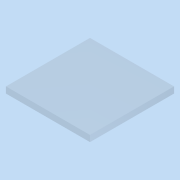
# Autodesk Inventor part: camera_hole_filter
Saved by Autodesk Inventor 2014 SP1 (Build 180222100, 222)
## iProperties
Created: 2013-03-31
Material: Glass
Document SubType Name: Modeling
Designer: Robert Davis
Mass: 1.35891 g
Surface Area: 13.4657 cm^2
Volume: 0.623352 cm^3
Density: 2.18 g/cm^3
Description: IR FILTER
Appearance: Clear - Light
Author: Robert Davis
Autodesk Inventor part; units mm, degrees
ref_plane "YZ Plane" through (0, 0, 0) normal (1, 0, 0) x (0, 1, 0)
sketch "Sketch1" plane through (0, 0, 0) normal (0, 0, 1) x (1, 0, 0)
  line L0 (0, 8.1841) -> (0, 0)
  line L1 (0, 0) -> (9.8567, 0)
  line L2 (-7.5, 7.5) -> (7.5, 7.5)
  line L3 (7.5, 7.5) -> (7.5, -7.5)
  line L4 (7.5, -7.5) -> (-7.5, -7.5)
  line L5 (-7.5, -7.5) -> (-7.5, 7.5)
  dimension "d0" = 15
  dimension "d1" = 15
  constraints: 12 end point, 2 horizontal, 1 coincident, 1 parallel, 1 vertical, 2 other
  measures "d0" distance of L2.start L2.end
  measures "d1" distance of L2.end L3.end
extrude "Extrusion1" add sketch "Sketch1" along normal mid plane 1.1
ref_plane "Work Plane1" through (-7.5, -7.5, 0) normal (0.7071, -0.7071, 0) x (0, 0, -1)
ref_plane "Work Plane2" through (7.5, -7.5, 0) normal (0.7071, 0.7071, 0) x (0, 0, -1)
body "Solid1"
